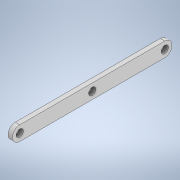
# Autodesk Inventor part: foot
Saved by Autodesk Inventor 2020 (Build 240168000, 168)
## iProperties
Created: 2019-12-21
Part Number: foot
Material: Générique
Document SubType Name: Modeling
Designer: damien
Density: 1 g/cm^3
Appearance: Par défaut
Author: damien
Autodesk Inventor part; units mm, degrees
ref_plane "YZ Plane" through (0, 0, 0) normal (1, 0, 0) x (0, 1, 0)
ref_plane "XZ Plane" through (0, 0, 0) normal (0, 1, 0) x (-1, 0, 0)
ref_plane "XY Plane" through (0, 0, 0) normal (0, 0, 1) x (1, 0, 0)
sketch "Esquisse1" plane through (0, 0, 0) normal (1, 0, 0) x (0, 1, 0)
  line L0 (-30, 330) -> (30, 330)
  line L1 (30, 330) -> (30, -330)
  line L2 (30, -330) -> (-30, -330)
  line L3 (-30, -330) -> (-30, 330)
  line L4 (-30, 330) -> (30, -330) construction
  line L5 (30, 330) -> (-30, -330) construction
  point P0 (0, 0)
  dimension "d0" = 660
  dimension "d1" = 60
  constraints: 12 end point, 2 midpoint, 2 parallel, 1 horizontal, 1 perpendicular
  measures "d0" distance of L0.end L1.end
  measures "d1" distance of L0.start L0.end
extrude "Extrusion1" add sketch "Esquisse1" along normal blind 18.55
sketch "Esquisse2" plane through (18.55, 0, 0) normal (1, 0, 0) x (0, 0, -1)
  circle A0 centre (-300, 0) radius 15
  circle A1 centre (0, 0) radius 15
  circle A2 centre (300, 0) radius 15
  line L0 (330, -30) -> (330, 30) projected
  line L1 (-330, 30) -> (-330, -30) projected
  line L2 (-330, 0) -> (330, 0) construction
  dimension "d4" = 30
  dimension "d5" = 30
  dimension "d6" = 30
  constraints: 3 centre point, 2 end point, 2 equal radius, 2 midpoint, 2 point on line, 1 coincident
  measures "d4" distance from line of L0 A2.centre
  measures "d5" diameter of A0
  measures "d6" distance from line of L1 A0.centre
extrude "Extrusion2" cut sketch "Esquisse2" against normal blind 18.55
fillet "Congé1" radius 30 1 edges at (9.275, 30, 330)
fillet "Congé2" radius 30 3 edges at (9.275, -30, 330) (9.275, 30, -330) (9.275, -30, -330)
